Autodesk Fusion 360 part; units mm, degrees
(part 2 of 2)
sketch "Sketch8" plane through (0, 0, 0) normal (0, 0, 1) x (1, 0, 0)
  circle A0 centre (49.4911, 7.1157) radius 1.55
  circle A1 centre (-37.7875, 32.743) radius 1.55
  circle A2 centre (0, -50) radius 1.55
  circle A3 centre (-49.4911, 7.1157) radius 1.55
  circle A4 centre (37.7875, 32.743) radius 1.55
  circle A5 centre (45.4816, -20.7708) radius 1.55
  circle A6 centre (-14.0866, 47.9746) radius 1.55
  circle A7 centre (-27.032, -42.0627) radius 1.55
  circle A8 centre (-45.4816, -20.7708) radius 1.55
  circle A9 centre (14.0866, 47.9746) radius 1.55
  circle A10 centre (27.032, -42.0627) radius 1.55
  circle A11 centre (0, 32.5) radius 2.55
  circle A12 centre (0, 0) radius 9.6
  circle A13 centre (-28.1458, 16.25) radius 2.55
  circle A14 centre (28.1458, 16.25) radius 2.55
  circle A15 centre (0, -32.5) radius 2.55
  circle A16 centre (-28.1458, -16.25) radius 2.55
  circle A17 centre (28.1458, -16.25) radius 2.55
  arc A18 (59.7646, 5.3101) -> (58.8397, 11.7426) centre (0, 0) ccw
  arc A19 (58.8397, 11.7426) -> (54.6515, 13.8844) centre (55.8977, 11.1555) ccw
  line L0 (54.6515, 13.8844) -> (44.1121, 9.0712)
  line L1 (44.1121, 9.0712) -> (35.7428, 27.3974)
  line L2 (35.7428, 27.3974) -> (46.2822, 32.2105)
  arc A20 (46.2822, 32.2105) -> (47.4063, 36.7783) centre (45.036, 34.9394) ccw
  arc A21 (47.4063, 36.7783) -> (43.1506, 41.6896) centre (0, 0) ccw
  arc A22 (43.1506, 41.6896) -> (38.4693, 41.2271) centre (40.9931, 39.6052) ccw
  line L3 (38.4693, 41.2271) -> (32.2052, 31.48)
  line L4 (32.2052, 31.48) -> (15.2567, 42.3722)
  line L5 (15.2567, 42.3722) -> (21.5207, 52.1193)
  arc A23 (21.5207, 52.1193) -> (19.9968, 56.5697) centre (18.997, 53.7412) ccw
  arc A24 (19.9968, 56.5697) -> (13.7615, 58.4005) centre (0, 0) ccw
  arc A25 (13.7615, 58.4005) -> (10.0734, 55.4805) centre (13.0734, 55.4805) ccw
  line L6 (10.0734, 55.4805) -> (10.0734, 43.8941)
  line L7 (10.0734, 43.8941) -> (-10.0734, 43.8941)
  line L8 (-10.0734, 43.8941) -> (-10.0734, 55.4805)
  arc A26 (-10.0734, 55.4805) -> (-13.7615, 58.4005) centre (-13.0734, 55.4805) ccw
  arc A27 (-13.7615, 58.4005) -> (-19.9968, 56.5697) centre (0, 0) ccw
  arc A28 (-19.9968, 56.5697) -> (-21.5207, 52.1193) centre (-18.997, 53.7412) ccw
  line L9 (-21.5207, 52.1193) -> (-15.2567, 42.3722)
  line L10 (-15.2567, 42.3722) -> (-32.2052, 31.48)
  line L11 (-32.2052, 31.48) -> (-38.4693, 41.2271)
  arc A29 (-38.4693, 41.2271) -> (-43.1506, 41.6896) centre (-40.9931, 39.6052) ccw
  arc A30 (-43.1506, 41.6896) -> (-47.4063, 36.7783) centre (0, 0) ccw
  arc A31 (-47.4063, 36.7783) -> (-46.2822, 32.2105) centre (-45.036, 34.9394) ccw
  line L12 (-46.2822, 32.2105) -> (-35.7428, 27.3974)
  line L13 (-35.7428, 27.3974) -> (-44.1121, 9.0712)
  line L14 (-44.1121, 9.0712) -> (-54.6515, 13.8844)
  arc A32 (-54.6515, 13.8844) -> (-58.8397, 11.7426) centre (-55.8977, 11.1555) ccw
  arc A33 (-58.8397, 11.7426) -> (-59.7646, 5.3101) centre (0, 0) ccw
  arc A34 (-59.7646, 5.3101) -> (-56.3494, 2.0752) centre (-56.7763, 5.0446) ccw
  line L15 (-56.3494, 2.0752) -> (-44.8809, 3.7241)
  line L16 (-44.8809, 3.7241) -> (-42.0137, -16.2176)
  line L17 (-42.0137, -16.2176) -> (-53.4822, -17.8666)
  arc A35 (-53.4822, -17.8666) -> (-55.8476, -21.9327) centre (-53.0553, -20.836) ccw
  arc A36 (-55.8476, -21.9327) -> (-53.148, -27.844) centre (0, 0) ccw
  arc A37 (-53.148, -27.844) -> (-48.526, -28.719) centre (-50.4906, -26.4518) ccw
  line L18 (-48.526, -28.719) -> (-39.7696, -21.1316)
  line L19 (-39.7696, -21.1316) -> (-26.5763, -36.3575)
  line L20 (-26.5763, -36.3575) -> (-35.3327, -43.945)
  arc A38 (-35.3327, -43.945) -> (-35.1243, -48.6444) centre (-33.3681, -46.2122) ccw
  arc A39 (-35.1243, -48.6444) -> (-29.6574, -52.1578) centre (0, 0) ccw
  arc A40 (-29.6574, -52.1578) -> (-25.296, -50.3952) centre (-28.1745, -49.55) ccw
  line L21 (-25.296, -50.3952) -> (-22.0318, -39.2781)
  line L22 (-22.0318, -39.2781) -> (-2.701, -44.9541)
  line L23 (-2.701, -44.9541) -> (-5.9653, -56.0712)
  arc A41 (-5.9653, -56.0712) -> (-3.2493, -59.912) centre (-3.0868, -56.9164) ccw
  arc A42 (-3.2493, -59.912) -> (3.2493, -59.912) centre (0, 0) ccw
  arc A43 (3.2493, -59.912) -> (5.9653, -56.0712) centre (3.0868, -56.9164) ccw
  line L24 (5.9653, -56.0712) -> (2.701, -44.9541)
  line L25 (2.701, -44.9541) -> (22.0318, -39.2781)
  line L26 (22.0318, -39.2781) -> (25.296, -50.3952)
  arc A44 (25.296, -50.3952) -> (29.6574, -52.1578) centre (28.1745, -49.55) ccw
  arc A45 (29.6574, -52.1578) -> (35.1243, -48.6444) centre (0, 0) ccw
  arc A46 (35.1243, -48.6444) -> (35.3327, -43.945) centre (33.3681, -46.2122) ccw
  line L27 (35.3327, -43.945) -> (26.5763, -36.3575)
  line L28 (26.5763, -36.3575) -> (39.7696, -21.1316)
  line L29 (39.7696, -21.1316) -> (48.526, -28.719)
  arc A47 (48.526, -28.719) -> (53.148, -27.844) centre (50.4906, -26.4518) ccw
  arc A48 (53.148, -27.844) -> (55.8476, -21.9327) centre (0, 0) ccw
  arc A49 (55.8476, -21.9327) -> (53.4822, -17.8666) centre (53.0553, -20.836) ccw
  line L30 (53.4822, -17.8666) -> (42.0137, -16.2176)
  line L31 (42.0137, -16.2176) -> (44.8809, 3.7241)
  line L32 (44.8809, 3.7241) -> (56.3494, 2.0752)
  arc A50 (56.3494, 2.0752) -> (59.7646, 5.3101) centre (56.7763, 5.0446) ccw
  circle A51 centre (0, 0) radius 14
  circle A52 centre (14, 0) radius 2.55
  circle A53 centre (0, 14) radius 2.55
  circle A54 centre (-14, 0) radius 2.55
  circle A55 centre (0, -14) radius 2.55
  dimension "d25" = 28
  dimension "d26" = 5.1
  dimension "d28" = 360
  constraint coincident A12.centre A18.centre
  constraint coincident A51 A52.centre
  measures "d25" diameter of A51
  measures "d26" diameter of A52
extrude "Extrude7" cut sketch "Sketch8" against normal blind 16 contours A51 A52 | A51 A52 | A51 A53 | A51 A53 | A51 A55 | A51 A55 | A51 A54 | A51 A54
